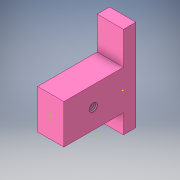
# Autodesk Inventor part: vexTempConnectionToCylinder
Saved by Autodesk Inventor 2016 SP1 (Build 200210100, 210)
## iProperties
Created: 2015-07-13
Part Number: vexTempConnectionToCylinder
Material: Aluminum 6061
Document SubType Name: Modeling
Designer: steele
Density: 2.7 g/cm^3
Appearance: Pink
Mass: 94.7579 g
Surface Area: 105.47 cm^2
Volume: 35.0955 cm^3
Author: steele
Autodesk Inventor part; units mm, degrees
ref_plane "YZ Plane" through (0, 0, 0) normal (1, 0, 0) x (0, 1, 0)
ref_plane "XZ Plane" through (0, 0, 0) normal (0, 1, 0) x (-1, 0, 0)
ref_plane "XY Plane" through (0, 0, 0) normal (0, 0, 1) x (1, 0, 0)
sketch "Sketch1" plane through (0, 0, 0) normal (0, 0, 1) x (1, 0, 0)
  line L0 (-6.35, -25.4) -> (6.35, -25.4)
  line L1 (6.35, -25.4) -> (6.35, 25.4)
  line L2 (6.35, 25.4) -> (-6.35, 25.4)
  line L3 (-6.35, 25.4) -> (-6.35, -25.4)
  line L4 (-6.35, -25.4) -> (6.35, 25.4) construction
  line L5 (6.35, -25.4) -> (-6.35, 25.4) construction
  point P0 (0, 0)
  dimension "height" = 50.8
  dimension "width" = 12.7
  constraints: 12 end point, 2 midpoint, 2 parallel, 1 horizontal, 1 perpendicular
  measures "height" distance of L0.end L1.end
  measures "width" distance of L1.end L2.end
extrude "Extrusion1" add sketch "Sketch1" against normal blind 12.7
sketch "Sketch3" plane through (0, 0, 0) normal (0, 0, 1) x (1, 0, 0)
  line L0 (-6.35, -9.525) -> (6.35, -9.525)
  line L1 (6.35, -9.525) -> (6.35, 9.525)
  line L2 (6.35, 9.525) -> (-6.35, 9.525)
  line L3 (-6.35, 9.525) -> (-6.35, -9.525)
  line L4 (-6.35, -9.525) -> (6.35, 9.525) construction
  line L5 (6.35, -9.525) -> (-6.35, 9.525) construction
  line L6 (6.35, 25.4) -> (-6.35, 25.4) projected
  point P0 (0, 0)
  dimension "Channel_Width" = 19.05
  dimension "d52" = 12.7
  constraints: 12 end point, 3 parallel, 2 midpoint, 1 perpendicular
  measures "Channel_Width" distance of L1.end L0.end
  measures "d52" distance of L1.end L2.end
extrude "Extrusion3" add sketch "Sketch3" along normal blind 28.448
sketch "Sketch6" plane through (6.35, -25.4, -12.7) normal (1, 0, 0) x (0, 0, -1)
  line L0 (-12.7, 25.4) -> (-41.148, 25.4) construction
  line L1 (-41.148, 15.875) -> (-41.148, 34.925) construction
  line L2 (-12.7, 34.925) -> (-12.7, 50.8) construction
  point P0 (-26.924, 25.4)
  dimension "d53" = 14.224
  constraints: 2 end point, 2 midpoint
  measures "d53" distance from line of point (-26.924, 25.4) L2
hole "Hole5" at (6.35, 0, 14.224) direction (-1, 0, 0) diameter 3.9624 end through all thread size "10-32 UNF" class "2B" standard "ANSI Unified Screw Threads"
sketch "Sketch13" plane through (6.35, -25.4, -12.7) normal (1, 0, 0) x (0, 0, -1)
  line L0 (-12.7, 50.8) -> (0, 50.8) projected
  line L1 (0, 0) -> (-6.35, 0)
  line L2 (-6.35, 0) -> (-6.35, 50.8)
  line L3 (-6.35, 50.8) -> (0, 50.8)
  line L4 (0, 50.8) -> (0, 0)
  point P0 (-12.7, 25.4)
  dimension "d98" = 6.35
  constraints: 8 end point, 2 parallel, 1 horizontal, 1 midpoint, 1 perpendicular
  measures "d98" distance between parallel lines of L2 L4
extrude "Extrusion5" cut sketch "Sketch13" against normal through all
sketch "Sketch14" plane through (-6.35, -25.4, 0) normal (-1, 0, 0) x (0, 0, 1)
  line L0 (0, 0) -> (-6.35, 0) projected
  line L1 (0, 0) -> (0, 15.875) projected
  line L2 (-6.35, 0) -> (0, 0)
  line L3 (0, 0) -> (0, 6.604)
  line L4 (0, 6.604) -> (-6.35, 6.604)
  line L5 (-6.35, 6.604) -> (-6.35, 0)
  point P0 (0, 25.4)
  dimension "d101" = 6.604
  constraints: 8 end point, 2 parallel, 1 horizontal, 1 perpendicular, 1 point on line
  measures "d101" distance of L3.end L2.end
extrude "Extrusion6" cut sketch "Sketch14" against normal through all
sketch "Sketch16" plane through (6.35, 9.525, 0) normal (1, 0, 0) x (0, 0, -1)
  point P0 (0, -9.525)
sketch "Sketch17" plane through (0, 0, 0) normal (0, 0, 1) x (1, 0, 0)
  line L0 (-6.35, 25.4) -> (-6.35, 9.525) projected
  line L1 (-6.35, 9.525) -> (6.35, 9.525) projected
  line L2 (-6.35, 25.4) -> (6.35, 25.4)
  line L3 (6.35, 25.4) -> (6.35, 9.525)
  line L4 (6.35, 9.525) -> (-6.35, 9.525)
  line L5 (-6.35, 9.525) -> (-6.35, 25.4)
  point P0 (0, 0)
  constraints: 8 end point, 2 parallel, 1 horizontal, 1 perpendicular
extrude "Extrusion7" cut sketch "Sketch17" against normal blind 0.381
sketch "Sketch18" plane through (0, 0, 0) normal (0, 0, 1) x (1, 0, 0)
  line L0 (-6.35, -18.796) -> (6.35, -18.796) projected
  line L1 (6.35, -9.525) -> (6.35, 9.525) projected
  line L2 (-6.35, -18.796) -> (6.35, -18.796)
  line L3 (6.35, -18.796) -> (6.35, -9.525)
  line L4 (6.35, -9.525) -> (-6.35, -9.525)
  line L5 (-6.35, -9.525) -> (-6.35, -18.796)
  point P0 (0, 0)
  constraints: 8 end point, 2 parallel, 1 horizontal, 1 perpendicular
extrude "Extrusion8" cut sketch "Sketch18" against normal blind 0.381
sketch "Sketch10" plane through (0, 0, 28.448) normal (0, 0, 1) x (1, 0, 0)
  point P0 (0, 0)
sketch "Sketch12" plane through (-6.35, -9.525, 0) normal (0, -1, 0) x (1, 0, 0)
  point P0 (15.875, 15.875)
equation "\"width\" = partWidth"
equation "\"d52\" = width"
equation "\"Channel_Height\" = 2 * centerLineOfCylinder"
equation "\"d53\" = centerLineOfCylinder"
equation "\"partWidth\" = 12.7"
equation "\"centerLineOfCylinder\" = 14.224"
body "Solid1"
